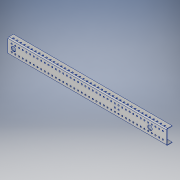
# Autodesk Inventor part: Side arm outer
Saved by Autodesk Inventor 2019 (Build 230136000, 136)
## iProperties
Created: 2018-11-07
Part Number: Side arm outer
Material: Aluminum 6061
Document SubType Name: Sheet Metal
Designer: woodk
Density: 2.7 g/cm^3
Sheet Metal Rule: Haakon
Appearance: Aluminum - Flat
Mass: 227.471 g
Surface Area: 907.912 cm^2
Volume: 84.2484 cm^3
Author: woodk
Autodesk Inventor part; units mm, degrees
ref_plane "YZ Plane" through (0, 0, 0) normal (1, 0, 0) x (0, 1, 0)
ref_plane "XZ Plane" through (0, 0, 0) normal (0, 1, 0) x (-1, 0, 0)
ref_plane "XY Plane" through (0, 0, 0) normal (0, 0, 1) x (1, 0, 0)
sketch "Sketch1" plane through (0, 0, 0) normal (0, 0, 1) x (1, 0, 0)
  line L0 (0, 0) -> (546.1, 0)
  line L1 (546.1, 0) -> (546.1, 50.8)
  line L2 (546.1, 50.8) -> (0, 50.8)
  line L3 (0, 50.8) -> (0, 0)
  dimension "d0" = 50.8
  dimension "d1" = 546.1
  measures "d0" distance of L2.end L0.start
  measures "d1" distance of L0.start L0.end
extrude "Plate1" add sketch "Sketch1" along normal blind 2.032
sketch "Sketch2" plane through (546.1, 48.768, 2.032) normal (0, 1, 0) x (-1, 0, 0)
  line L0 (546.1, 0) -> (0, 0)
  line L1 (0, 0) -> (0, -19.05)
  line L2 (0, -19.05) -> (546.1, -19.05)
  line L3 (546.1, -19.05) -> (546.1, 0)
  constraints: 6 end point, 1 horizontal, 1 perpendicular, 1 vertical
edge flange "Flange1" height 19.05 angle 90 thickness 2.032 bend radius 1.27 thickness toward (0, 1, 0) relief tear relief width 2.032 relief depth 1.016 edges at (273.05, 50.8, 0) wall of the first edge with corners at (0, 48.768, 2.032) (546.1, 48.768, 2.032) (546.1, 48.768, -17.018) (0, 48.768, -17.018)
bend "Bend1"
corner "Corner1"
sketch "Sketch3" plane through (0, 2.032, 2.032) normal (0, -1, 0) x (1, 0, 0)
  line L0 (546.1, 0) -> (0, 0)
  line L1 (0, 0) -> (0, -19.05)
  line L2 (0, -19.05) -> (546.1, -19.05)
  line L3 (546.1, -19.05) -> (546.1, 0)
  constraints: 6 end point, 1 horizontal, 1 perpendicular, 1 vertical
edge flange "Flange2" height 19.05 angle 90 thickness 2.032 bend radius 1.27 thickness toward (0, -1, 0) relief tear relief width 2.032 relief depth 1.016 edges at (273.05, 0, 0) wall of the first edge with corners at (546.1, 2.032, 2.032) (0, 2.032, 2.032) (0, 2.032, -17.018) (546.1, 2.032, -17.018)
bend "Bend2"
corner "Corner2"
sketch "Sketch4" plane through (0, 0, 2.032) normal (0, 0, 1) x (1, 0, 0)
  line L0 (0, 3.302) -> (0, 47.498) projected
  line L1 (0, 50.8) -> (546.1, 50.8) projected
  line L2 (546.1, 0) -> (0, 0) projected
  point P0 (12.7, 38.1)
  point P1 (12.7, 12.7)
  dimension "d23" = 12.7
  dimension "d24" = 12.7
  dimension "d25" = 12.7
  constraints: 1 vertical alignment
  measures "d23" distance from line of L0 point (12.7, 38.1)
  measures "d24" distance from line of L1 point (12.7, 38.1)
  measures "d25" distance from line of L2 point (12.7, 12.7)
hole "Hole1" at (12.7, 38.1, 2.032) at (12.7, 12.7, 2.032) direction (0, 0, -1) diameter 4.9784 end through all
pattern_linear "Rectangular Pattern1" count 42 spacing 12.7 along (1, 0, 0) of "Hole1"
sketch "Sketch5" plane through (0, 50.8, -17.018) normal (0, 1, 0) x (1, 0, 0)
  line L0 (546.1, -19.05) -> (0, -19.05) projected
  line L1 (0, -15.748) -> (0, 0) projected
  point P0 (0, -17.018)
  point P1 (12.7, -12.7)
  dimension "d36" = 6.35
  dimension "d37" = 12.7
  measures "d36" distance from line of L0 point (12.7, -12.7)
  measures "d37" distance from line of L1 point (12.7, -12.7)
hole "Hole2" at (12.7, 50.8, -4.318) direction (0, -1, 0) diameter 4.9784 end through all
pattern_linear "Rectangular Pattern2" count 42 spacing 12.7 along (1, 0, 0) of "Hole2"
sketch "Sketch6" plane through (0, 0, 2.032) normal (0, 0, 1) x (1, 0, 0)
  line L0 (546.1, 47.498) -> (546.1, 3.302) projected
  point P0 (0, 0)
  point P1 (488.95, 25.4)
  point P2 (546.1, 25.4)
  dimension "d48" = 57.15
  constraints: 1 horizontal alignment, 1 midpoint
  measures "d48" distance from line of L0 point (488.95, 25.4)
hole "Hole3" at (488.95, 25.4, 2.032) direction (0, 0, -1) diameter 15.875 end through all
sketch "Sketch7" plane through (0, 0, 2.032) normal (0, 0, 1) x (1, 0, 0)
  line L0 (546.1, 47.498) -> (546.1, 3.302) projected
  point P0 (0, 0)
  point P1 (368.3, 25.4)
  point P2 (381, 25.4)
  point P3 (546.1, 25.4)
  dimension "d56" = 12.7
  dimension "d57" = 165.1
  constraints: 2 horizontal alignment, 1 midpoint
  measures "d56" distance of point (368.3, 25.4) point (381, 25.4)
  measures "d57" distance from line of L0 point (381, 25.4)
hole "Hole4" at (368.3, 25.4, 2.032) at (381, 25.4, 2.032) direction (0, 0, -1) diameter 4.9784 end through all
sketch "Sketch8" plane through (0, 0, 2.032) normal (0, 0, 1) x (1, 0, 0)
  line L0 (0, 3.302) -> (0, 47.498) projected
  point P0 (0, 0)
  point P1 (19.05, 25.4)
  point P2 (0, 25.4)
  dimension "d65" = 19.05
  constraints: 1 horizontal alignment, 1 midpoint
  measures "d65" distance from line of L0 point (19.05, 25.4)
hole "Hole5" at (19.05, 25.4, 2.032) direction (0, 0, -1) diameter 15.875 end through all
equation "\"d31\" = Thickness"
equation "\"d43\" = Thickness"
equation "\"d54\" = Thickness"
equation "\"d63\" = Thickness"
equation "\"d71\" = Thickness"
equation "\"d2\" = Thickness"
equation "\"d3\" = BendReliefWidth"
equation "\"d4\" = BendReliefDepth"
equation "\"d5\" = MinimumRemnant"
equation "\"d6\" = TransitionRadius"
equation "\"d9\" = BendRadius"
equation "\"d10\" = CornerReliefSize"
equation "\"d11\" = GapSize"
equation "\"d12\" = JacobiRadiusSize"
equation "\"d13\" = BendReliefWidth"
equation "\"d14\" = BendReliefDepth"
equation "\"d15\" = MinimumRemnant"
equation "\"d16\" = TransitionRadius"
equation "\"d19\" = BendRadius"
equation "\"d20\" = CornerReliefSize"
equation "\"d21\" = GapSize"
equation "\"d22\" = JacobiRadiusSize"
equation "\"BendReliefWidth\" = Thickness"
equation "\"BendReliefDepth\" = 0.5 * Thickness"
equation "\"CornerReliefSize\" = 4 * Thickness"
equation "\"MinimumRemnant\" = 2 * Thickness"
equation "\"TransitionRadius\" = BendRadius"
equation "\"JacobiRadiusSize\" = BendRadius"
equation "\"GapSize\" = Thickness"
equation "\"Thickness\" = 2.032"
equation "\"BendRadius\" = 1.27"
body "Solid1"
